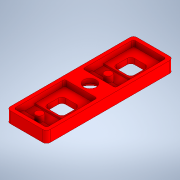
# Autodesk Inventor part: LineSensorPlate
Saved by Autodesk Inventor 2021 (Build 250183000, 183)
## iProperties
Created: 2022-02-28
Part Number: LineSensorPlate
Material: Generic
Document SubType Name: Modeling
Designer: ermoz
Density: 1 g/cm^3
Appearance: Default
Author: ermoz
Autodesk Inventor part; units mm, degrees
ref_plane "YZ Plane" through (0, 0, 0) normal (1, 0, 0) x (0, 1, 0)
ref_plane "XZ Plane" through (0, 0, 0) normal (0, 1, 0) x (-1, 0, 0)
ref_plane "XY Plane" through (0, 0, 0) normal (0, 0, 1) x (1, 0, 0)
sketch "Sketch1" plane through (0, 0, 0) normal (0, 1, 0) x (-1, 0, 0)
  line L0 (0, 0) -> (8, 0)
  line L1 (8, 0) -> (8, -13)
  line L2 (8, -13) -> (0, -13)
  line L3 (0, -13) -> (0, 0)
  line L4 (8.5, -13.5) -> (8.5, 0.5)
  line L5 (8.5, 0.5) -> (-0.5, 0.5)
  line L6 (-0.5, 0.5) -> (-0.5, -13.5)
  line L7 (-0.5, -13.5) -> (8.5, -13.5)
  line L8 (0, -19) -> (8, -19)
  line L9 (8, -19) -> (8, -32)
  line L10 (8, -32) -> (0, -32)
  line L11 (0, -32) -> (0, -19)
  line L12 (8.5, -32.5) -> (8.5, -18.5)
  line L13 (8.5, -18.5) -> (-0.5, -18.5)
  line L14 (-0.5, -18.5) -> (-0.5, -32.5)
  line L15 (-0.5, -32.5) -> (8.5, -32.5)
  line L16 (9.5, 1.5) -> (-1.5, 1.5)
  line L17 (-1.5, 1.5) -> (-1.5, -33.5)
  line L18 (-1.5, -33.5) -> (9.5, -33.5)
  line L19 (9.5, -33.5) -> (9.5, 1.5)
  circle A0 centre (4, -16) radius 1.75
  line L20 (4, -18.5) -> (4, -13.5)
  dimension "d0" = 8
  dimension "d1" = 13
  dimension "d2" = 0.5
  dimension "d3" = 0.5
  dimension "d4" = 3.5
  dimension "d5" = 2.5
  dimension "d6" = 2.5
  dimension "d7" = 1
  dimension "d8" = 1
  dimension "d9" = 1
  dimension "d10" = 1
  constraints: 42 end point, 10 parallel, 5 perpendicular, 3 horizontal, 3 midpoint, 2 equal length, 1 centre point, 1 collinear, 6 other
  measures "d0" distance of L1.end L2.end
  measures "d1" distance of L0.end L1.end
  measures "d2" distance between parallel lines of L1 L4
  measures "d3" distance between parallel lines of L9 L12
  measures "d4" diameter of A0
  measures "d5" distance from line of L7 A0.centre
  measures "d6" distance from line of L13 A0.centre
  measures "d7" distance between parallel lines of L16 L5
  measures "d8" distance between parallel lines of L18 L15
  measures "d9" distance between parallel lines of L19 L12
  measures "d10" distance between parallel lines of L17 L14
extrude "Extrusion1" add sketch "Sketch1" along normal blind 1.6 contours L19 L18 L17 L16
sketch "Sketch2" plane through (0, 0, 0) normal (0, -1, 0) x (1, 0, 0)
  line L0 (-9.5, 1.5) -> (1.5, 1.5) projected
  line L1 (1.5, -33.5) -> (-9.5, -33.5) projected
  line L2 (1.5, 1.5) -> (-9.5, 1.5)
  line L3 (-9.5, 1.5) -> (-9.5, -33.5)
  line L4 (-9.5, -33.5) -> (1.5, -33.5)
  line L5 (1.5, -33.5) -> (1.5, 1.5)
  circle A0 centre (-4, -16) radius 1.75 projected
  circle A1 centre (-4, -16) radius 1.75
  line L6 (-1.5, -24.75) -> (-6.5, -24.75)
  line L7 (-6.5, -24.75) -> (-6.5, -29.75)
  line L8 (-6.5, -29.75) -> (-1.5, -29.75)
  line L9 (-1.5, -29.75) -> (-1.5, -24.75)
  line L10 (-1.5, -5.75) -> (-6.5, -5.75)
  line L11 (-6.5, -5.75) -> (-6.5, -10.75)
  line L12 (-6.5, -10.75) -> (-1.5, -10.75)
  line L13 (-1.5, -10.75) -> (-1.5, -5.75)
  line L14 (-8.5, -18.5) -> (-8.5, -32.5) projected
  line L15 (-8.5, -32.5) -> (0.5, -32.5) projected
  line L16 (0.5, -18.5) -> (-8.5, -18.5) projected
  line L17 (-4, -18.5) -> (-4, -23.5281)
  line L18 (-8.5, -13.5) -> (0.5, -13.5) projected
  point P0 (0, 0)
  dimension "d14" = 5
  dimension "d15" = 2.75
  dimension "d16" = 5
  dimension "d17" = 2.75
  constraints: 26 end point, 6 parallel, 3 horizontal, 3 perpendicular, 2 collinear, 1 centre point, 1 coincident, 1 midpoint, 1 point on line, 1 vertical, 1 other
  measures "d14" distance of L6.start L6.end
  measures "d15" distance between parallel lines of L15 L8
  measures "d16" distance of L8.end L6.start
  measures "d17" distance between parallel lines of L12 L18
extrude "Extrusion2" add sketch "Sketch2" along normal blind 1.5
sketch "Sketch3" plane through (0, 0, 0) normal (0, 1, 0) x (1, 0, 0)
  circle A0 centre (-4, 2) radius 1
  circle A1 centre (-4, 21) radius 1
  line L0 (0.5, 18.5) -> (-8.5, 18.5) projected
  circle A2 centre (-4, 16) radius 1.75 projected
  line L1 (0.5, -0.5) -> (-8.5, -0.5) projected
  point P0 (0, 0)
  dimension "d20" = 2.5
  dimension "d21" = 2.5
  dimension "d22" = 2
  constraints: 2 centre point, 2 vertical alignment, 1 equal radius
  measures "d20" distance from line of L0 A1.centre
  measures "d21" distance from line of L1 A0.centre
  measures "d22" diameter of A1
extrude "Extrusion3" add sketch "Sketch3" along normal blind 1.5 contours A0 | A1
chamfer "Chamfer1" distance 2 angle 45 1 edges at (-5.75, -1.5, -16)
fillet "Fillet1" radius 1 4 edges at (-9.5, 0.05, 1.5) (1.5, 0.05, 1.5) (-9.5, 0.05, -33.5) (1.5, 0.05, -33.5)
fillet "Fillet2" radius 1 8 edges at (-6.5, -0.75, -5.75) (-1.5, -0.75, -5.75) (-1.5, -0.75, -10.75) (-6.5, -0.75, -10.75) (-6.5, -0.75, -24.75) (-1.5, -0.75, -24.75) (-1.5, -0.75, -29.75) (-6.5, -0.75, -29.75)
fillet "Fillet3" radius 0.5 8 edges at (0.5, 0.8, -32.5) (-8.5, 0.8, -32.5) (-8.5, 0.8, -18.5) (0.5, 0.8, -18.5) (0.5, 0.8, -13.5) (-8.5, 0.8, -13.5) (-8.5, 0.8, 0.5) (0.5, 0.8, 0.5)
sketch "Sketch4" plane through (0, 0, 0) normal (0, 1, 0) x (1, 0, 0)
  line L0 (-8.5, 24.25) -> (0.5, 24.25)
  line L1 (0.5, 24.25) -> (0.5, 21)
  line L2 (0.5, 21) -> (-8.5, 21)
  line L3 (-8.5, 21) -> (-8.5, 24.25)
  line L4 (-8.5, 5.25) -> (0.5, 5.25)
  line L5 (0.5, 5.25) -> (0.5, 2)
  line L6 (0.5, 2) -> (-8.5, 2)
  line L7 (-8.5, 2) -> (-8.5, 5.25)
  line L8 (-8.5, 19) -> (-8.5, 32) projected
  line L9 (0.5, 32) -> (0.5, 19) projected
  line L10 (-5.5, 24.75) -> (-2.5, 24.75) projected
  circle A0 centre (-4, 21) radius 1 projected
  circle A1 centre (-4, 2) radius 1 projected
  line L11 (-5.5, 5.75) -> (-2.5, 5.75) projected
  point P0 (0, 0)
  point P1 (-5, 2)
  point P2 (-3, 2)
  point P3 (-5, 21)
  point P4 (-3, 21)
  dimension "d32" = 0.5
  dimension "d34" = 0.5
  constraints: 16 end point, 4 collinear, 4 parallel, 2 horizontal, 2 midpoint, 2 perpendicular
  measures "d32" distance between parallel lines of L10 L0
  measures "d34" distance between parallel lines of L11 L4
extrude "Extrusion4" cut sketch "Sketch4" against normal blind 0.5 contours L0 L1 L2 A0 L3 | L4 L5 L6 A1 L7
equation "\"d3\" = d2"
equation "\"d6\" = d5"
equation "\"d8\" = d7"
equation "\"d10\" = d9"
equation "\"d17\" = d15"
equation "\"d21\" = d20"
equation "\"d34\" = d32"
body "Solid1"
